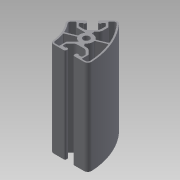
# Autodesk Inventor part: 40-4094
Saved by Autodesk Inventor 2013 (Build 170138000, 138)
## iProperties
Created: 2014-04-23
Part Number: 40-4094
Material: Generic
Document SubType Name: Modeling
Designer: Ross Bowman
Density: 1 g/cm^3
Engineer: Ross Bowman
Catalog Web Link: 8020.net
Vendor: 80/20 Inc.
Company: 80/20 Inc.
Author: Ross Bowman
Keywords: 80/20 , 8020 , T-Slot , Extrusion
Material: 6105-T5 Aluminum
Autodesk Inventor part; units mm, degrees
ref_plane "YZ Plane" through (0, 0, 0) normal (1, 0, 0) x (0, 1, 0)
ref_plane "XZ Plane" through (0, 0, 0) normal (0, 1, 0) x (-1, 0, 0)
ref_plane "XY Plane" through (0, 0, 0) normal (0, 0, 1) x (1, 0, 0)
sketch "Sketch1" plane through (0, 0, 0) normal (0, 0, 1) x (1, 0, 0)
  line L0 (-14.1673, 14.7841) -> (-14.8136, 15.4308)
  arc A0 (-14.8136, 15.4308) -> (-17.0404, 15.4314) centre (-15.9273, 14.3177) ccw
  arc A1 (-14.168, 12.5572) -> (-14.1673, 14.7841) centre (-15.281, 13.671) ccw
  line L1 (-17.0404, 15.4314) -> (-24.4856, 7.9907)
  line L2 (-14.6677, 12.0578) -> (-14.168, 12.5572)
  arc A2 (-24.4856, 7.9907) -> (-24.7333, 2.6036) centre (-21.658, 5.1614) ccw
  arc A3 (-15.1955, 12.0488) -> (-14.6677, 12.0578) centre (-14.9362, 12.3266) ccw
  arc A4 (-15.6538, -19.3255) -> (-24.7333, 2.6036) centre (-55.4871, -22.9739) ccw
  line L3 (-15.2163, 12.0682) -> (-15.1955, 12.0488)
  arc A5 (-15.6538, -19.3255) -> (-11.6705, -22.9607) centre (-11.6705, -18.9607) ccw
  arc A6 (-15.2163, 12.0682) -> (-15.7441, 12.0592) centre (-15.4755, 11.7904) ccw
  line L4 (-11.6705, -22.9607) -> (-1.1445, -22.9607)
  line L5 (-17.0957, 10.7084) -> (-15.7441, 12.0592)
  arc A7 (-1.1445, -22.9607) -> (0.4301, -21.3861) centre (-1.1445, -21.3861) ccw
  arc A8 (-17.0957, 10.7084) -> (-17.0962, 8.9126) centre (-16.198, 9.8102) ccw
  line L6 (0.4301, -21.3861) -> (0.4301, -20.4718)
  line L7 (-15.3713, 7.1867) -> (-17.0962, 8.9126)
  arc A9 (0.4301, -20.4718) -> (-1.1445, -18.8972) centre (-1.1445, -20.4718) ccw
  arc A10 (-15.3713, 7.1867) -> (-14.7429, 6.9261) centre (-14.7426, 7.815) ccw
  line L8 (-1.1445, -18.8972) -> (-1.851, -18.8972)
  line L9 (-10.0952, 6.9247) -> (-14.7429, 6.9261)
  arc A11 (-1.851, -18.8972) -> (-2.2307, -19.2639) centre (-1.851, -19.2772) ccw
  arc A12 (-10.0952, 6.9247) -> (-6.7366, 8.3148) centre (-10.0938, 11.674) ccw
  line L10 (-2.2307, -19.2639) -> (-2.2317, -19.2924)
  line L11 (-1.954, 13.0945) -> (-6.7366, 8.3148)
  arc A13 (-2.6115, -19.6591) -> (-2.2317, -19.2924) centre (-2.6115, -19.2792) ccw
  arc A14 (-1.954, 13.0945) -> (-0.562, 16.4523) centre (-5.3112, 16.4537) ccw
  line L12 (-2.6115, -19.6591) -> (-4.5223, -19.6591)
  line L13 (-0.5607, 21.0999) -> (-0.562, 16.4523)
  arc A15 (-5.7922, -18.3893) -> (-4.5223, -19.6591) centre (-4.5223, -18.3893) ccw
  arc A16 (-0.5607, 21.0999) -> (-0.8208, 21.7286) centre (-1.4496, 21.1002) ccw
  line L14 (-5.7922, -18.3893) -> (-5.7922, -15.9492)
  line L15 (-2.5457, 23.4545) -> (-0.8208, 21.7286)
  arc A17 (-5.5318, -15.3207) -> (-5.7922, -15.9492) centre (-4.9033, -15.9492) ccw
  arc A18 (-2.5457, 23.4545) -> (-4.3416, 23.455) centre (-3.4439, 22.5568) ccw
  line L16 (-5.5318, -15.3207) -> (-2.2454, -12.0343)
  line L17 (-5.6931, 22.1042) -> (-4.3416, 23.455)
  arc A19 (1.1128, -10.6433) -> (-2.2454, -12.0343) centre (1.1128, -15.3925) ccw
  arc A20 (-5.6931, 22.1042) -> (-5.7025, 21.5764) centre (-5.4246, 21.8355) ccw
  line L18 (1.1128, -10.6433) -> (7.8743, -10.6433)
  line L19 (-5.6831, 21.5555) -> (-5.7025, 21.5764)
  arc A21 (11.2325, -12.0343) -> (7.8743, -10.6433) centre (7.8743, -15.3925) ccw
  arc A22 (-5.6924, 21.0278) -> (-5.6831, 21.5555) centre (-5.961, 21.2965) ccw
  line L20 (11.2325, -12.0343) -> (14.5189, -15.3207)
  line L21 (-6.237, 20.4835) -> (-5.6924, 21.0278)
  arc A23 (14.7793, -15.9492) -> (14.5189, -15.3207) centre (13.8904, -15.9492) ccw
  arc A24 (-8.4127, 20.5227) -> (-6.237, 20.4835) centre (-7.3047, 21.6219) ccw
  line L22 (14.7793, -15.9492) -> (14.7793, -18.3893)
  line L23 (-9.059, 21.1694) -> (-8.4127, 20.5227)
  arc A25 (13.5094, -19.6591) -> (14.7793, -18.3893) centre (13.5094, -18.3893) ccw
  arc A26 (-9.1095, 23.3576) -> (-9.059, 21.1694) centre (-7.9264, 22.2903) ccw
  line L24 (13.5094, -19.6591) -> (11.5986, -19.6591)
  line L25 (-1.7967, 30.6661) -> (-9.1095, 23.3576)
  arc A27 (11.2188, -19.2924) -> (11.5986, -19.6591) centre (11.5986, -19.2792) ccw
  arc A28 (4.0055, 30.5111) -> (-1.7967, 30.6661) centre (1.0309, 27.8368) ccw
  line L26 (11.2188, -19.2924) -> (11.2179, -19.2639)
  arc A29 (24.4013, -18.7495) -> (4.0055, 30.5111) centre (-55.4871, -22.9739) ccw
  arc A30 (11.2179, -19.2639) -> (10.8381, -18.8972) centre (10.8381, -19.2772) ccw
  arc A31 (20.4069, -22.9607) -> (24.4013, -18.7495) centre (20.4069, -18.9607) ccw
  line L27 (10.8381, -18.8972) -> (10.0682, -18.8972)
  line L28 (10.0682, -22.9607) -> (20.4069, -22.9607)
  arc A32 (10.0682, -18.8972) -> (8.5571, -20.4629) centre (10.1178, -20.4572) ccw
  arc A33 (8.5571, -21.3772) -> (10.0682, -22.9607) centre (10.1505, -21.3694) ccw
  line L29 (8.5571, -20.4629) -> (8.5571, -21.3772)
  line L30 (1.5037, 21.6586) -> (-2.9893, 26.1515)
  arc A34 (-2.9891, 27.2265) -> (-2.9893, 26.1515) centre (-2.4519, 26.6889) ccw
  arc A35 (1.7262, 21.1212) -> (1.5037, 21.6586) centre (0.9662, 21.1212) ccw
  line L31 (-2.9891, 27.2265) -> (-0.6647, 29.5496)
  line L32 (1.7262, 15.9317) -> (1.7262, 21.1212)
  arc A36 (2.7429, 29.4599) -> (-0.6647, 29.5496) centre (0.9966, 27.8874) ccw
  arc A37 (0.0375, 11.8546) -> (1.7262, 15.9317) centre (-4.0396, 15.9317) ccw
  arc A38 (16.2826, 8.4768) -> (2.7429, 29.4599) centre (-55.4871, -22.9739) ccw
  line L33 (-1.5568, 10.2604) -> (0.0375, 11.8546)
  arc A39 (15.8773, 7.4696) -> (16.2826, 8.4768) centre (15.5865, 8.1717) ccw
  arc A40 (-1.5568, 10.2604) -> (-1.7668, 9.5852) centre (-1.0194, 9.723) ccw
  line L34 (15.8773, 7.4696) -> (6.6079, 3.6301)
  line L35 (-1.3792, 7.4825) -> (-1.7668, 9.5852)
  arc A41 (5.8356, 3.866) -> (6.6079, 3.6301) centre (6.3649, 4.2167) ccw
  arc A42 (-1.3792, 7.4825) -> (-0.692, 6.9657) centre (-0.7547, 7.5976) ccw
  arc A43 (5.8356, 3.866) -> (-0.692, 6.9657) centre (0, 0) ccw
  arc A44 (22.7652, -18.8985) -> (17.5072, 5.5193) centre (-55.4871, -22.9739) ccw
  arc A45 (20.4184, -21.3707) -> (22.7652, -18.8985) centre (20.4184, -19.0207) ccw
  arc A46 (17.5072, 5.5193) -> (16.5084, 5.945) centre (16.7993, 5.2429) ccw
  line L36 (20.4184, -21.3707) -> (17.1382, -21.3707)
  line L37 (7.2394, 2.1057) -> (16.5084, 5.945)
  arc A47 (16.3782, -20.6107) -> (17.1382, -21.3707) centre (17.1382, -20.6107) ccw
  arc A48 (7.2394, 2.1057) -> (6.8601, 1.3927) centre (7.4824, 1.519) ccw
  line L38 (16.3782, -20.6107) -> (16.3782, -14.2517)
  arc A49 (4.4362, -5.4148) -> (6.8601, 1.3927) centre (0, 0) ccw
  arc A50 (16.3782, -14.2517) -> (16.1556, -13.7143) centre (15.6182, -14.2517) ccw
  arc A51 (4.4362, -5.4148) -> (4.3157, -6.2662) centre (4.8387, -5.906) ccw
  line L39 (16.1556, -13.7143) -> (12.486, -10.0448)
  line L40 (5.5285, -8.0271) -> (4.3157, -6.2662)
  arc A52 (12.486, -10.0448) -> (8.409, -8.356) centre (8.409, -14.1218) ccw
  arc A53 (5.5285, -8.0271) -> (6.1544, -8.356) centre (6.1544, -7.596) ccw
  line L41 (8.409, -8.356) -> (6.1544, -8.356)
  circle A54 centre (0, 0) radius 3.3782
  line L42 (-7.3708, -14.2314) -> (-7.3708, -20.6107)
  arc A55 (-8.1308, -21.3707) -> (-7.3708, -20.6107) centre (-8.1308, -20.6107) ccw
  arc A56 (-7.1482, -13.694) -> (-7.3708, -14.2314) centre (-6.6108, -14.2314) ccw
  line L43 (-8.1308, -21.3707) -> (-11.6733, -21.3707)
  line L44 (-1.3284, -7.8742) -> (-7.1482, -13.694)
  arc A57 (-14.0138, -19.2319) -> (-11.6733, -21.3707) centre (-11.6733, -19.0207) ccw
  arc A58 (-1.3284, -7.8742) -> (-1.6296, -6.8077) centre (-1.7774, -7.4252) ccw
  arc A59 (-14.0138, -19.2319) -> (-16.4433, -8.4957) centre (-55.4871, -22.9739) ccw
  arc A60 (-5.8356, -3.866) -> (-1.6296, -6.8077) centre (0, 0) ccw
  arc A61 (-16.0216, -7.5293) -> (-16.4433, -8.4957) centre (-15.7307, -8.2315) ccw
  arc A62 (-5.8356, -3.866) -> (-6.6079, -3.6301) centre (-6.3649, -4.2167) ccw
  line L45 (-16.0216, -7.5293) -> (-6.6079, -3.6301)
  line L46 (-23.3636, 6.864) -> (-20.8622, 9.3639)
  arc A63 (-19.7876, 9.3638) -> (-20.8622, 9.3639) centre (-20.325, 8.8264) ccw
  arc A64 (-23.3636, 6.864) -> (-23.5072, 3.6967) centre (-21.7024, 5.2018) ccw
  line L47 (-19.7876, 9.3638) -> (-15.275, 4.8512)
  arc A65 (-17.6341, -5.6193) -> (-23.5072, 3.6967) centre (-55.4871, -22.9739) ccw
  arc A66 (-15.275, 4.8512) -> (-14.7376, 4.6286) centre (-14.7376, 5.3886) ccw
  arc A67 (-17.6341, -5.6193) -> (-16.6524, -6.0047) centre (-16.9432, -5.3025) ccw
  line L48 (-14.7376, 4.6286) -> (-6.5073, 4.6286)
  line L49 (-7.2394, -2.1057) -> (-16.6524, -6.0047)
  arc A68 (-5.966, 3.6615) -> (-6.5073, 4.6286) centre (-6.5073, 3.9936) ccw
  arc A69 (-5.966, 3.6615) -> (-6.8601, -1.3927) centre (0, 0) ccw
  arc A70 (-7.2394, -2.1057) -> (-6.8601, -1.3927) centre (-7.4824, -1.519) ccw
  constraints: 140 point on circle, 100 end point, 71 centre point
extrude "Extrusion1" add sketch "Sketch1" against normal blind 100
body "Solid1"
